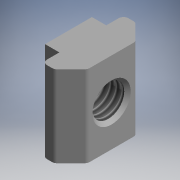
# Autodesk Inventor part: HNTT8-8
Saved by Autodesk Inventor 2017.3 (Build 213256000, 256)
## iProperties
Part Number: HNTT8-8
Material: Generic
Catalog Web Link: www.cadenas.de
Description: HNTT8, HNTTV8, HNTTZ8, HNTTSN8, HNTTSS8-Pre-Assembly Insertion Nuts for Aluminum Extrusions - Standard -HFS8 Series (Aluminum Extrusions 40, 80 Square)-
Vendor: MISUMI
Document SubType Name: Modeling
Designer: partserver
Manufacturer: MISUMI
Mass: 1.69428 g
Surface Area: 11.3722 cm^2
Volume: 1.69428 cm^3
Density: 1 g/cm^3
Appearance: PSOLRGB-192-192-192
Category: PARTsolutions
Company: MISUMI
Title: HNTT8-8
Author: Cadenas PARTsolutions
Comments: Pre-Assembly Insertion Nuts for Aluminum Extrusions - Standard -HFS8 Series (Aluminum Extrusions 40, 80 Square)-
PSOL_IDENT_0: {$CADENAS_DATA\23d-libs\misumi\metric\38_al_extrusions_blackets\nuts\hntt8.prj},188 {VTYP=3D},{NB=HN
PSOL_IDENT_1: TT8-8},{LINA=HNTT8-8},{NN=HNTT8, HNTTV8, HNTTZ8, HNTTSN8, HNTTSS8},{DATE=08.06.2021 08:27:46},{GEOMD
PSOL_IDENT_2: ATE=31.10.2014 05:13:00},{VERSION=},{LINEID=40},{WBVAR=M},{WBNUMERIC=}  {NB=HNTT8-8},{LINA=HNTT8-8},
PSOL_IDENT_3: {KT=DUMMY},{PN=HNTT8-8},{TYPE=HNTT8},{MAT=1010 Carbon Steel Equivalent},{M=8},{MALG= '4' , '5' , '6'
PSOL_IDENT_4: , '8' },{M3D=8},{A=9.8},{B=17.0},{E=6.0},{T=9.0},{L=17},{TT=10},{TAPER=3.500}
NB: HNTT8-8
NN: HNTT8, HNTTV8, HNTTZ8, HNTTSN8, HNTTSS8
NT: Pre-Assembly Insertion Nuts for Aluminum Extrusions - Standard -HFS8 Series (Aluminum Extrusions 40, 80 Square)-
NBSYN: $PN.
LINA: HNTT8-8
CATALOG: Misumi
PN: HNTT8-8
MAT: 1010 Carbon Steel Equivalent
M: 8
SUPPLIER: MISUMI
ARTICLENO: HNTT8-8
BOMINFO: HNTT8-8
CREATOR: CADENAS GmbH
Autodesk Inventor part; units mm, degrees
sketch "Sketch_1" plane through (0, 0, 0) normal (0, 0, 1) x (1, 0, 0)
  arc A0 (-9, -4.5858) -> (-8.7071, -5.2929) centre (-8, -4.5858) ccw
  line L0 (-8.7071, -5.2929) -> (-5.7929, -8.2071)
  arc A1 (-5.7929, -8.2071) -> (-5.0858, -8.5) centre (-5.0858, -7.5) ccw
  line L1 (-5.0858, -8.5) -> (-4, -8.5)
  arc A2 (-4, -8.5) -> (-3, -7.5) centre (-4, -7.5) ccw
  line L2 (-3, -7.5) -> (-3, -4.9)
  line L3 (-3, -4.9) -> (0, -4.9)
  line L4 (0, -4.9) -> (0, 4.9)
  line L5 (0, 4.9) -> (-3, 4.9)
  line L6 (-3, 4.9) -> (-3, 7.5)
  arc A3 (-3, 7.5) -> (-4, 8.5) centre (-4, 7.5) ccw
  line L7 (-4, 8.5) -> (-5.0858, 8.5)
  arc A4 (-5.0858, 8.5) -> (-5.7929, 8.2071) centre (-5.0858, 7.5) ccw
  line L8 (-5.7929, 8.2071) -> (-8.7071, 5.2929)
  arc A5 (-8.7071, 5.2929) -> (-9, 4.5858) centre (-8, 4.5858) ccw
  line L9 (-9, 4.5858) -> (-9, -4.5858)
  constraints: 20 end point, 12 point on circle, 6 centre point
extrude "Extrusion1" add sketch "Sketch_1" along normal mid plane 17
sketch "Sketch_5" plane through (0, 0, 0) normal (0, 0, 1) x (1, 0, 0)
  line L0 (0, 0) -> (-9, 0)
  line L1 (-9, 0) -> (-9, 4)
  line L2 (-9, 4) -> (-8.3235, 3.3235)
  line L3 (-8.3235, 3.3235) -> (-0.6765, 3.3235)
  line L4 (-0.6765, 3.3235) -> (0, 4)
  line L5 (0, 4) -> (0, 0)
  line L6 (0, 0) -> (-9, 0)
  constraints: 14 end point
revolve "Revolution1" cut sketch "Sketch_5" angle 360 about axis through (0, 0, 0) along (1, 0, 0)
thread "Thread1" size "M8x1.25" class "6H" standard "ISO Metric profile" full length
ref_plane "nut_XY" through (0, 0, 0) normal (1, 0, 0) x (0, 0, -1)
ref_plane "nut_YZ" through (0, 0, 0) normal (0, 0, -1) x (0, 1, 0)
ref_plane "nut_ZX" through (0, 0, 0) normal (0, 1, 0) x (1, 0, 0)
ref_plane "to_bolt_XY" through (-9, 0, 0) normal (1, 0, 0) x (0, 0, -1)
ref_plane "to_bolt_YZ" through (-9, 0, 0) normal (0, 0, -1) x (0, 1, 0)
ref_plane "to_bolt_ZX" through (-9, 0, 0) normal (0, 1, 0) x (1, 0, 0)
ref_plane "to_frames_XY" through (-3, 0, 0) normal (1, 0, 0) x (0, 0, -1)
ref_plane "to_frames_YZ" through (-3, 0, 0) normal (0, 0, -1) x (0, 1, 0)
ref_plane "to_frames_ZX" through (-3, 0, 0) normal (0, 1, 0) x (1, 0, 0)
body "Solid1"
